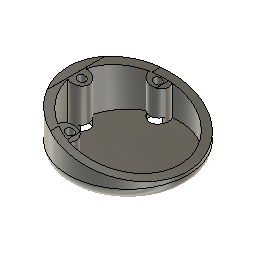
CapUR_link2 (Autodesk Fusion 360 design; units mm, degrees)
part number: 2025-04-09-17-50-51-443
Autodesk Fusion 360 part; units mm, degrees
note: some values were not read from the file. Set by a fixed rule: which sketch regions a step uses.
sketch "Sketch1" plane through (0, 0, 0) normal (0, 0, 1) x (1, 0, 0)
  circle A0 centre (0, 0) radius 38.1
  circle A1 centre (0, 0) radius 33.1
  dimension "d1" = 76.2
  dimension "d2" = 5
  constraint coincident A0.centre A1.centre
  constraint concentric A0 A1
  measures "d1" diameter of A0
  measures "d2" distance of A0 A1
extrude "Extrude1" add sketch "Sketch1" along normal blind 60
ref_plane "WorkPlane1" through (0, -70, 0) normal (0, 1, 0) x (0, 0, 1)
sketch "Sketch2" plane through (0, -70, 0) normal (0, 1, 0) x (1, 0, 0)
  line L0 (-38.1, -30) -> (38.1, -10)
  line L1 (-38.1, -30) -> (-38.1, -60)
  line L2 (-38.1, -60) -> (38.1, -60)
  line L3 (38.1, -60) -> (38.1, -10)
  constraint perpendicular L1 L2
  constraint perpendicular L2 L3
extrude "Extrude2" cut sketch "Sketch2" along normal blind 140
extrude "Extrude3" add sketch "Sketch1" along normal blind 2 contours A1
fillet "Fillet1" radius 8 1 edges at (-35.5217, -13.7775, 0)
sketch "Sketch3" plane through (0, 0, 2) normal (0, 0, 1) x (-1, 0, 0)
  circle A0 centre (0, 0) radius 33.1
  circle A1 centre (31, 0) radius 6
  circle A2 centre (29.55, 0) radius 2.5
  circle A3 centre (9.5795, 29.4828) radius 6
  circle A4 centre (9.1315, 28.1037) radius 2.5
  circle A5 centre (9.5795, -29.4828) radius 6
  circle A6 centre (9.1315, -28.1037) radius 2.5
  dimension "d31" = 12
  dimension "d32" = 5
  dimension "d33" = 1.45
  dimension "d35" = 360
  measures "d31" diameter of A1
  measures "d32" diameter of A2
  measures "d33" distance of A1.centre A2.centre
extrude "Extrude4" add sketch "Sketch3" along normal blind 27.19 contours A0 A1 | A0 A3 | A0 A5 picked at (31.3936, -4.0644) picked at (6.8367, 31.622) picked at (6.8367, -31.622)
sketch "Sketch4" plane through (0, -70, 0) normal (0, 1, 0) x (1, 0, 0)
  line L0 (-14.4896, -23.8029) -> (-14.4896, -24)
  line L1 (-14.4896, -24) -> (-7, -24)
  line L2 (-7, -24) -> (-6.4, -24)
  line L3 (-6.4, -24) -> (-6.4, -21.7)
  line L4 (-6.4, -21.7) -> (-14.4896, -23.8029)
  line L5 (-14.4896, -23.8029) -> (-33.3157, -28.6969)
  line L6 (-33.3157, -28.6969) -> (-33.3157, -29.5)
  line L7 (-33.3157, -29.5) -> (-3, -29.5)
  line L8 (-3, -29.5) -> (-3, -20.8126)
  line L9 (-6.4, -21.7) -> (-3, -20.8126)
  constraint vertical L0
  constraint perpendicular L0 L1
  constraint parallel L1 L2
  constraint perpendicular L1 L3
  constraint parallel L4 L5
  constraint perpendicular L1 L6
  constraint perpendicular L0 L7
  constraint perpendicular L7 L8
extrude "Extrude6" cut sketch "Sketch4" along normal blind 140
extrude "Extrude7" cut sketch "Sketch3" against normal blind 25 contours A2 | A4 | A6
sketch "Sketch5" plane through (0, 0, 0) normal (0, 0, -1) x (1, 0, 0)
  arc A0 (-11.6092, 27.7711) -> (-6.9314, 29.2911) centre (-9.1315, 28.1037) ccw
  arc A1 (-11.6092, 27.7711) -> (-29.9994, 2.4593) centre (0, 0) ccw
  arc A2 (-29.9994, -2.4593) -> (-29.9994, 2.4593) centre (-29.55, 0) ccw
  arc A3 (-29.9994, -2.4593) -> (-11.6092, -27.7711) centre (0, 0) ccw
  arc A4 (-6.9314, -29.2911) -> (-11.6092, -27.7711) centre (-9.1315, -28.1037) ccw
  arc A5 (-6.9314, -29.2911) -> (-6.9314, 29.2911) centre (0, 0) ccw
  circle A6 centre (-9.1315, 28.1037) radius 5
  circle A7 centre (-29.55, 0) radius 5
  circle A8 centre (-9.1315, -28.1037) radius 5
  dimension "d36" = 10
  dimension "d37" = 10
  dimension "d38" = 10
  constraint concentric A0 A6
  constraint concentric A2 A7
  constraint concentric A4 A8
  measures "d36" diameter of A6
  measures "d37" diameter of A7
  measures "d38" diameter of A8
extrude "Extrude8" cut sketch "Sketch5" against normal blind 5.2 contours A0 A1 A5 A6 | A0 A1 A5 A6 | A1 A2 A3 A7 | A1 A2 A3 A7 | A3 A4 A5 A8 | A3 A4 A5 A8
